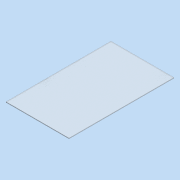
# Autodesk Inventor part: Floor
Saved by Autodesk Inventor 2016 SP1 (Build 200210100, 210)
## iProperties
Created: 2015-11-19
Part Number: Floor
Material: Acrylic, Clear
Document SubType Name: Modeling
Designer: Mohamed A.
Density: 1.19 g/cm^3
Appearance: Transparent - Clear
Mass: 535.5 g
Surface Area: 3048 cm^2
Volume: 450 cm^3
Author: Mohamed A.
Autodesk Inventor part; units mm, degrees
ref_plane "YZ Plane" through (0, 0, 0) normal (1, 0, 0) x (0, 1, 0)
ref_plane "XZ Plane" through (0, 0, 0) normal (0, 1, 0) x (-1, 0, 0)
ref_plane "XY Plane" through (0, 0, 0) normal (0, 0, 1) x (1, 0, 0)
sketch "Sketch1" plane through (0, 0, 0) normal (0, 0, 1) x (1, 0, 0)
  line L0 (150, 250) -> (-150, 250)
  line L1 (-150, 250) -> (-150, -250)
  line L2 (-150, -250) -> (150, -250)
  line L3 (150, -250) -> (150, 250)
  line L4 (150, 250) -> (-150, -250) construction
  line L5 (-150, 250) -> (150, -250) construction
  point P0 (0, 0)
  dimension "d0" = 300
  dimension "d1" = 500
  constraints: 12 end point, 2 midpoint, 2 parallel, 1 horizontal, 1 perpendicular
  measures "d0" distance of L2.end L1.end
  measures "d1" distance of L1.end L0.end
extrude "Extrusion1" add sketch "Sketch1" along normal blind 3
sketch "Sketch4" plane through (0, 0, 3) normal (0, 0, 1) x (1, 0, 0)
  line L0 (-105.1666, -140.2454) -> (-24.9469, -94.301) construction
  line L1 (-23.8333, -140.2454) -> (-105.9352, -95.7824) construction
  point P0 (0, 0)
  point P1 (-23.8333, -96.2454)
  point P2 (-105.1666, -96.2454)
  point P3 (-38.8284, -102.2514)
  point P4 (-91.4635, -103.6196)
  point P5 (-91.4635, -132.3972)
  point P6 (-38.3251, -132.3972)
  constraints: 4 end point, 4 point on line, 4 other
hole "Hole3" [suppressed]
body "Solid1"
